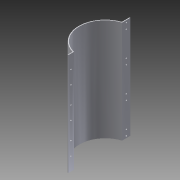
# Autodesk Inventor part: 装填斗罩
Saved by Autodesk Inventor 2015 (Build 190159000, 159)
## iProperties
Created: 2017-05-04
Part Number: 装填斗罩
Material: 常规
Document SubType Name: Modeling
Designer: Administrator
Density: 1 g/cm^3
Appearance: 雪
Author: Administrator
Autodesk Inventor part; units mm, degrees
ref_plane "YZ Plane" through (0, 0, 0) normal (1, 0, 0) x (0, 1, 0)
ref_plane "XZ Plane" through (0, 0, 0) normal (0, 1, 0) x (-1, 0, 0)
ref_plane "XY Plane" through (0, 0, 0) normal (0, 0, 1) x (1, 0, 0)
sketch "草图1" plane through (0, 0, 0) normal (0, 0, 1) x (1, 0, 0)
  circle A0 centre (0, 0) radius 100
  line L0 (-25, -96.8246) -> (25, -96.8246)
  line L1 (25, -96.8246) -> (25, -118)
  line L2 (25, -118) -> (-25, -118)
  line L3 (-25, -118) -> (-25, -96.8246)
  arc A1 (-33, 97.5705) -> (-28, -99.1211) centre (0, 0) ccw
  line L4 (-28, -118) -> (-28, -99.1211)
  line L5 (-28, -118) -> (-25, -118)
  line L6 (-30, 95.3939) -> (-30, 127.5705)
  line L7 (-30, 127.5705) -> (-33, 127.5705)
  line L8 (-33, 127.5705) -> (-33, 97.5705)
  line L9 (0, -100) -> (25, -100)
  dimension "d0" = 200
  dimension "d2" = 50
  dimension "d3" = 33
  dimension "d4" = 3
  dimension "d5" = 3
  dimension "d6" = 3
  dimension "d7" = 30
  dimension "d10" = 18
  constraints: 20 end point, 6 point on circle, 4 perpendicular, 2 centre point, 2 horizontal, 2 parallel, 2 vertical, 1 coincident, 1 concentric, 1 point on line, 1 tangent
  measures "d0" diameter of A0
  measures "d2" distance of L1.end L2.end
  measures "d3" horizontal distance of point (0, 0) L8.end
  measures "d4" radial gap between concentric circles of A1 A0
  measures "d5" distance between parallel lines of L3 L4
  measures "d6" distance of L6.end L7.end
  measures "d7" distance of L7.end L8.end
  measures "d10" distance between parallel lines of L2 L9
extrude "拉伸1" add sketch "草图1" against normal blind 398 contours A0 L3 L5 L4 A1 L8 L7 L6
sketch "草图2" plane through (-28, -118, 0) normal (-1, 0, 0) x (0, 0, 1)
  circle A0 centre (-53, 10) radius 2.5
  circle A1 centre (-105, 10) radius 2.5
  line L0 (0, 18.8789) -> (0, 0) projected
  line L1 (0, 0) -> (-398, 0) projected
  point P0 (0, 118)
  dimension "d11" = 5
  dimension "d12" = 5
  dimension "d13" = 53
  dimension "d14" = 105
  dimension "d15" = 10
  dimension "d16" = 10
  constraints: 2 centre point
  measures "d11" diameter of A0
  measures "d12" diameter of A1
  measures "d13" distance from line of L0 A0.centre
  measures "d14" distance from line of L0 A1.centre
  measures "d15" distance from line of L1 A0.centre
  measures "d16" distance from line of L1 A1.centre
extrude "拉伸2" cut sketch "草图2" against normal blind 3
pattern_linear "矩形阵列1" count 3 spacing 120 along (0, 0, -1) of "拉伸2"
sketch "草图3" plane through (-33, 97.5705, 0) normal (-1, 0, 0) x (0, 0, 1)
  circle A0 centre (-8, 15) radius 2.5
  circle A1 centre (-30, 15) radius 2.5
  line L0 (0, 30) -> (0, 0) projected
  line L1 (0, 30) -> (-398, 30) projected
  point P0 (0, -97.5705)
  dimension "d22" = 5
  dimension "d23" = 5
  dimension "d24" = 8
  dimension "d25" = 30
  dimension "d26" = 15
  dimension "d27" = 15
  constraints: 2 centre point
  measures "d22" diameter of A0
  measures "d23" diameter of A1
  measures "d24" distance from line of L0 A0.centre
  measures "d25" distance from line of L0 A1.centre
  measures "d26" distance from line of L1 A0.centre
  measures "d27" distance from line of L1 A1.centre
extrude "拉伸3" cut sketch "草图3" against normal blind 3
pattern_linear "矩形阵列2" count 4 spacing 120 along (0, 0, -1) of "拉伸3"
